Autodesk Fusion 360 part; units mm, degrees
(part 4 of 4)
sketch "Sketch1 (2)" plane through (0, 0, 0) normal (0, 0, 1) x (1, 0, 0) in component "Watch Face Sheet"
  line L0 (30.097, 15.3359) -> (30.097, -17.6641)
  line L1 (60.097, 15.3359) -> (30.097, 15.3359)
  line L2 (60.097, -17.6641) -> (60.097, 15.3359)
  line L3 (30.097, -17.6641) -> (60.097, -17.6641)
  line L4 (26.197, 17.7359) -> (63.997, 17.7359)
  line L5 (63.997, 17.7359) -> (63.997, -20.0641)
  line L6 (63.997, -20.0641) -> (26.197, -20.0641)
  line L7 (26.197, -20.0641) -> (26.197, 17.7359)
  line L8 (30.097, -1.1641) -> (26.197, -1.1641) construction
  line L9 (63.997, -1.1641) -> (60.097, -1.1641) construction
  line L10 (45.097, 15.3359) -> (45.097, 17.7359) construction
  line L11 (45.097, -17.6641) -> (45.097, -20.0641) construction
  line L12 (28.597, 15.3359) -> (61.597, 15.3359)
  line L13 (61.597, 15.3359) -> (61.597, -17.6641)
  line L14 (61.597, -17.6641) -> (28.597, -17.6641)
  line L15 (28.597, -17.6641) -> (28.597, 15.3359)
  line L16 (28.597, 15.3359) -> (61.597, -17.6641) construction
  line L17 (61.597, 15.3359) -> (28.597, -17.6641) construction
  line L18 (30.097, 15.3359) -> (60.097, -17.6641) construction
  circle A0 centre (28.597, 15.3359) radius 0.8
  circle A1 centre (28.597, -17.6641) radius 0.8
  circle A2 centre (61.597, -17.6641) radius 0.8
  circle A3 centre (61.597, 15.3359) radius 0.8
  point P0 (45.097, -1.1641)
  point P1 (45.097, -1.1641)
  dimension "d53" = 37.8
  dimension "d54" = 37.8
  dimension "d131" = 33
  dimension "d132" = 33
  dimension "d133" = 1.6
  dimension "d134" = 1.6
  dimension "d135" = 1.6
  dimension "d136" = 1.6
  constraint horizontal L4
  constraint vertical L5
  constraint horizontal L6
  constraint vertical L7
  constraint midpoint L0 L8.start
  constraint midpoint L7 L8.end
  constraint midpoint L5 L9.start
  constraint midpoint L2 L9.end
  constraint midpoint L1 L10.start
  constraint midpoint L4 L10.end
  constraint midpoint L3 L11.start
  constraint midpoint L6 L11.end
  constraint vertical L11
  constraint horizontal L9
  constraint horizontal L12
  constraint perpendicular L12 L13
  constraint parallel L12 L14
  constraint parallel L13 L15
  constraint coincident L16 P1
  constraint coincident L17 P1
  constraint coincident L0.start L1.end
  constraint coincident L2.start L3.end
  constraint midpoint L18 P1
  constraint coincident P1 P0
  constraint coincident L12.start L15.end
  constraint coincident L14.end L15.start
  constraint coincident L13.end L14.start
  constraint coincident L12.end L13.start
  measures "d53" distance of L4.start L4.end
  measures "d54" distance of L4.start L6.end
  measures "d131" distance of L12.end L13.end
  measures "d132" distance of L12.start L12.end
  measures "d133" diameter of A0
  measures "d134" diameter of A1
  measures "d135" diameter of A2
  measures "d136" diameter of A3
extrude "Extrude1''''" add sketch "Sketch1" along normal blind 0.5 separate body makes body 15 in component "Watch Face Text"
extrude "Extrude1'''''" add sketch "Sketch1 (2)" along normal blind 0.5 separate body contours L0 L12 L14 L15 A0 A1 | L2 L12 L13 L14 A2 A3 | L4 L5 L6 L7 makes body 16 in component "Watch Face Sheet"
fillet "Fillet1''" radius 2 4 edges at (63.997, 17.7359, 0.25) (63.997, -20.0641, 0.25) (26.197, -20.0641, 0.25) (26.197, 17.7359, 0.25) on bodies 16 in component "Watch Face Sheet"
copy_body "CopyPasteBodies1" bodies 3 body 3 seen with x (0, 1, 0) y (0, 0, 1) z (1, 0, 0) at (18.6, -11, 4.8) makes body 17 in component "Button Plus Support"
move_body "Move1" bodies 17 to x (1, 0, 0) y (0, 1, 0) z (0, 0, 1) at (0, 0, 0) in component "Button Plus Support"
move_body "Move2" bodies 17 to x (1, 0, 0) y (0, 1, 0) z (0, 0, 1) at (-18.6, 11, -4.8) in component "Button Plus Support"
move_body "Move3" bodies 17 to x (0, 0, 1) y (0, 1, 0) z (-1, 0, 0) at (0, 0, 0) in component "Button Plus Support"
sketch "Wordy Watch Button with Support" plane through (0, 0, 0) normal (0, 0, 1) x (1, 0, 0) in component "Button Plus Support"
  line L0 (0.15, 5) -> (-0.15, 5)
  line L1 (-0.15, 5) -> (-0.15, -5)
  line L2 (-0.15, -5) -> (0.15, -5)
  line L3 (0.15, -5) -> (0.15, 5)
  line L4 (0.15, 5) -> (-0.15, -5) construction
  line L5 (-0.15, 5) -> (0.15, -5) construction
  circle A0 centre (0, 0) radius 5
  line L6 (1.75, 0.15) -> (5, 0.15)
  line L7 (5, 0.15) -> (5, -0.15)
  line L8 (5, -0.15) -> (1.75, -0.15)
  line L9 (1.75, -0.15) -> (1.75, 0.15)
  arc A1 (-1.3611, -1.1) -> (-1.3611, 1.1) centre (0, 0) ccw
  line L10 (0, 0) -> (1.75, 0) construction
  circle A2 centre (0, 0) radius 3
  point P0 (5, 0)
  point P1 (0, 5)
  point P2 (1.75, 0)
  dimension "d249" = 0.3
  dimension "d250" = 10
  dimension "d259" = 0.3
  dimension "d260" = -2
  constraint coincident A0.centre A1.centre
  constraint horizontal L0
  constraint perpendicular L0 L1
  constraint parallel L0 L2
  constraint parallel L1 L3
  constraint coincident L4 A0.centre
  constraint coincident L5 A0.centre
  constraint horizontal L6
  constraint vertical L7
  constraint horizontal L8
  constraint vertical L9
  constraint midpoint L7 P0
  constraint coincident A0 P0
  constraint midpoint A1 P2
  constraint coincident L9 P2
  constraint midpoint L0 P1
  constraint coincident A0 P1
  constraint midpoint L9 P2
  constraint coincident P2 L10.end
  measures "d249" distance of L1.end L2.end
  measures "d250" distance of L0.end L1.end
  measures "d259" distance of L6.start L8.end
extrude "Extrude1''''''" add sketch "Wordy Watch Button with Support" along normal blind 0.2 contours L1 L3 A0 A2 | L3 A0 L6 A2 | L1 A0 A2 | L1 L3 A1 A2 | A0 L6 L8 A2 | L1 L3 A0 A2 | L6 L8 L9 A2 | L1 L3 A1 A2 | L3 A0 L8 A2 bodies 17 in component "Button Plus Support"
chamfer "Chamfer1'" distance 0.5 angle 45 1 edges at (0.6328, -1.6316, 1) on bodies 17 in component "Button Plus Support"
component "LiPo Battery" placed x (1, 0, 0) y (0, -1, 0) z (0, 0, -1) at (3, 12.5, 4.05)
component "PCB" placed x (1, 0, 0) y (0, -1, 0) z (0, 0, -1) at (0, 0, 6.6)
component "Case Button" placed x (0, 1, 0) y (0, 0, 1) z (1, 0, 0) at (18.6, -11, 4.8)
component "WatchCase" placed x (1, 0, 0) y (0, 1, 0) z (0, 0, 1) at (0, 0, 0)
component "Watch Face Text" placed x (1, 0, 0) y (0, 1, 0) z (0, 0, 1) at (-45.097, 1.1641, 7.6)
component "Watch Face Sheet" placed x (1, 0, 0) y (0, 1, 0) z (0, 0, 1) at (-45.097, 1.1641, 7.6)
component "Button Plus Support" placed x (1, 0, 0) y (0, 1, 0) z (0, 0, 1) at (0, 0, 0)
equation "BatteryLength = 25 mm"
equation "BatteryWidth = 20 mm"
equation "BatteryHeight = 3.5 mm"
equation "d4 = BatteryWidth - BatteryHeight"
equation "BatteryRadius = 3 mm"
equation "d7 = BatteryHeight / 2"
equation "d9 = BatteryLength"
equation "CaseLength = 41 mm"
equation "CaseWidth = 41 mm"
equation "LugWidth = 20 mm"
equation "LugToBody = 3 mm"
equation "StrapPinDiameter = 1.8 mm"
equation "StrapPinEndDiam = 1 mm"
equation "CaseSideWall = 1.6 mm"
equation "FixingInset = 4 mm"
equation "FixingDiameter = 1.6 mm"
equation "FixingDiamTolerance = 0.4 mm"
equation "FixingBossDiam = FixingDiameter + 3 mm"
equation "d32 = CaseLength - 2 * FixingInset"
equation "d33 = CaseWidth - 2 * FixingInset"
equation "d34 = FixingDiamForSelfTap"
equation "d35 = FixingDiamForSelfTap"
equation "d36 = FixingDiamForSelfTap"
equation "d37 = FixingDiamForSelfTap"
equation "d38 = FixingBossDiam"
equation "d39 = FixingBossDiam"
equation "d40 = FixingBossDiam"
equation "d41 = FixingBossDiam"
equation "d42 = CaseWidth"
equation "d43 = CaseLength"
equation "d44 = CaseSideWall"
equation "WatchGlassWidth = 35 mm"
equation "WatchGlassHeight = 35 mm"
equation "WatchGlassThickness = 2 mm"
equation "d48 = WatchFaceThickness"
equation "WatchFaceWidth = CaseWidth - CaseSideWall * 2"
equation "WatchFaceLength = CaseLength - CaseSideWall * 2"
equation "WatchFaceThickness = 0.5 mm"
equation "d53 = WatchFaceWidth"
equation "d54 = WatchFaceLength"
equation "d55 = WatchFaceThickness"
equation "CaseBaseThickness = 1.3 mm"
equation "d62 = CaseBaseThickness"
equation "PCBLowCompHeight = 1 mm"
equation "d65 = BatteryHeight + PCBLowCompHeight"
equation "PCBThickness = 0.8 mm"
equation "LEDHeight = 1 mm"
equation "DiffuserThickness = 1 mm"
equation "CaseWallHeight = BatteryHeight + PCBLowCompHeight + PCBThickness + DiffuserThickness + WatchFaceThickness"
equation "d71 = CaseBaseThickness + CaseWallHeight"
equation "PCBWidth = 36 mm"
equation "PCBLength = 36 mm"
equation "d79 = PCBWidth"
equation "d80 = PCBLength"
equation "d99 = PCBThickness"
equation "d101 = PCBThickness + 2 mm"
equation "d103 = PCBThickness + 0.2 mm"
equation "d105 = PCBThickness + 3 mm"
equation "d131 = CaseWidth - 2 * FixingInset"
equation "d132 = CaseWidth - 2 * FixingInset"
equation "d133 = FixingDiameter"
equation "d134 = FixingDiameter"
equation "d135 = FixingDiameter"
equation "d136 = FixingDiameter"
equation "StrapFixWidth = 22 mm"
equation "StrapFlangeLength = 4 mm"
equation "StrapFlangeWidth = 6 mm"
equation "StrapFlangeDepth = 4 mm"
equation "d149 = StrapFlangeWidth"
equation "d150 = StrapFlangeLength"
equation "d151 = StrapFlangeWidth"
equation "d152 = StrapFlangeLength"
equation "d153 = StrapFixWidth / 2"
equation "d154 = StrapFixWidth / 2"
equation "d160 = -StrapFlangeDepth"
equation "d162 = StrapPinEndDiam"
equation "d164 = -StrapPinEndLen"
equation "d167 = StrapPinEndLen"
equation "StrapPinEndLen = 10 mm"
equation "d178 = CaseLength - FixingInset * 2"
equation "d179 = CaseWidth - FixingInset * 2"
equation "d180 = FixingDiameter"
equation "d181 = FixingDiameter"
equation "d182 = FixingDiameter"
equation "d183 = FixingDiameter"
equation "d189 = ( 4.8 * 0.4 ) * 1 mm"
equation "d191 = ( 4.8 * 0.4 ) * 1 mm"
equation "d193 = ( 4.8 * 0.4 ) * 1 mm"
equation "ButtonBackDiam = 3.5 mm"
equation "ButtonFrontDiam = 2 mm"
equation "ButtonBackDepth = 0.5 mm"
equation "ButtonDepthTotal = CaseSideWall + 1 mm"
equation "SwitchPegWidth = 1.9 mm"
equation "SwitchPegHeight = 0.8 mm"
equation "SwitchPegTolerance = 0.15 mm"
equation "d202 = SwitchPegHeight + SwitchPegTolerance * 2"
equation "d203 = SwitchPegWidth + SwitchPegTolerance * 2"
equation "d204 = ButtonBackDiam"
equation "d205 = ButtonFrontDiam"
equation "d206 = ButtonBackDepth"
equation "ButtonMidDepth = 0.5 mm"
equation "d210 = ButtonMidDepth"
equation "d213 = ButtonDepthTotal - ButtonBackDepth - ButtonMidDepth"
equation "d215 = ButtonFrontDiam + ButtonFitTolerance * 2"
equation "d216 = ButtonFrontDiam + ButtonFitTolerance * 2"
equation "ButtonFitTolerance = 0.2 mm"
equation "d218 = ButtonFrontDiam + ButtonFitTolerance * 2"
equation "d219 = ButtonBackDiam + ButtonFitTolerance * 2"
equation "d220 = ButtonBackDiam + ButtonFitTolerance * 2"
equation "d221 = ButtonBackDiam + ButtonFitTolerance * 2"
equation "d223 = ButtonMidDepth + ButtonFitTolerance"
equation "d226 = ButtonMidDepth + ButtonFitTolerance"
equation "d239 = 5 mm + ( 5.5 / 2 ) * 1 mm"
equation "FixingDiamForSelfTap = FixingDiameter - FixingDiamTolerance"
named bodies: "Text", "FaceSurround", "Wordy Watch Case", "PCB", "Wordy Watch Button", "Button (1)", "Button (2)", "Wordy Watch Button with Support"
